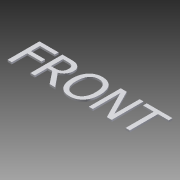
# Autodesk Inventor part: FrontLabel
Saved by Autodesk Inventor 2012 (Build 160160000, 160)
## iProperties
Created: 2014-07-21
Part Number: FrontLabel
Material: Default
Document SubType Name: Modeling
Designer: Anon
Density: 1 g/cm^3
Author: Anon
Autodesk Inventor part; units mm, degrees
ref_plane "YZ Plane" through (0, 0, 0) normal (1, 0, 0) x (0, 1, 0)
ref_plane "XZ Plane" through (0, 0, 0) normal (0, 1, 0) x (-1, 0, 0)
ref_plane "XY Plane" through (0, 0, 0) normal (0, 0, 1) x (1, 0, 0)
sketch "Sketch1" plane through (0, 0, 0) normal (0, 0, 1) x (1, 0, 0)
  line L0 (-12.3971, 6.4501) -> (24.1995, 6.4501) construction
  line L1 (24.1995, 6.4501) -> (24.1995, -12.763) construction
  line L2 (24.1995, -12.763) -> (-12.3971, -12.763) construction
  line L3 (-12.3971, -12.763) -> (-12.3971, 6.4501) construction
  line L4 (-9.9493, 5.9623) -> (-11.5774, 5.9623)
  line L5 (-11.5774, 5.9623) -> (-11.5774, 4.9753)
  line L6 (-11.5774, 4.9753) -> (-10.0174, 4.9753)
  line L7 (-10.0174, 4.9753) -> (-10.0174, 4.5612)
  line L8 (-10.0174, 4.5612) -> (-11.5774, 4.5612)
  line L9 (-11.5774, 4.5612) -> (-11.5774, 2.8764)
  line L10 (-11.5774, 2.8764) -> (-12.0425, 2.8764)
  line L11 (-12.0425, 2.8764) -> (-12.0425, 6.3764)
  line L12 (-12.0425, 6.3764) -> (-9.9493, 6.3764)
  line L13 (-9.9493, 6.3764) -> (-9.9493, 5.9623)
  line L14 (-6.8237, 2.8764) -> (-7.4279, 2.8764)
  line L15 (-7.4279, 2.8764) -> (-8.534, 4.269)
  line L16 (-8.534, 4.269) -> (-9.0673, 4.269)
  line L17 (-9.0673, 4.269) -> (-9.0673, 2.8764)
  line L18 (-9.0673, 2.8764) -> (-9.5324, 2.8764)
  line L19 (-9.5324, 2.8764) -> (-9.5324, 6.3764)
  line L20 (-9.5324, 6.3764) -> (-8.6305, 6.3764)
  spline S0 degree 2 poles (-8.6305, 6.3764) (-8.3298, 6.3764) (-7.9242, 6.3112) (-7.7399, 6.192) knots 0 0 0 1 2 2 2
  spline S1 degree 2 poles (-7.7399, 6.192) (-7.5555, 6.0729) (-7.3428, 5.7014) (-7.3428, 5.4262) knots 0 0 0 1 2 2 2
  spline S2 degree 2 poles (-7.3428, 5.4262) (-7.3428, 5.0433) (-7.7342, 4.5243) (-8.0689, 4.3995) knots 0 0 0 1 2 2 2
  line L21 (-8.0689, 4.3995) -> (-6.8237, 2.8764)
  spline S3 degree 2 poles (-7.8278, 5.3894) (-7.8278, 5.5425) (-7.9356, 5.7779) (-8.049, 5.8545) knots 0 0 0 1 2 2 2
  spline S4 degree 2 poles (-8.049, 5.8545) (-8.1483, 5.9197) (-8.4121, 5.9736) (-8.6049, 5.9736) knots 0 0 0 1 2 2 2
  line L22 (-8.6049, 5.9736) -> (-9.0673, 5.9736)
  line L23 (-9.0673, 5.9736) -> (-9.0673, 4.6576)
  line L24 (-9.0673, 4.6576) -> (-8.6588, 4.6576)
  spline S5 degree 2 poles (-8.6588, 4.6576) (-8.4574, 4.6576) (-8.1369, 4.7285) (-8.0263, 4.8391) knots 0 0 0 1 2 2 2
  spline S6 degree 2 poles (-8.0263, 4.8391) (-7.9242, 4.9356) (-7.8278, 5.2078) (-7.8278, 5.3894) knots 0 0 0 1 2 2 2
  spline S7 degree 2 poles (-4.0697, 5.9765) (-3.8711, 5.7439) (-3.6499, 5.0632) (-3.6499, 4.6264) knots 0 0 0 1 2 2 2
  spline S8 degree 2 poles (-3.6499, 4.6264) (-3.6499, 4.2009) (-3.8655, 3.5117) (-4.0697, 3.2791) knots 0 0 0 1 2 2 2
  spline S9 degree 2 poles (-4.0697, 3.2791) (-4.2852, 3.0352) (-4.8553, 2.8026) (-5.1985, 2.8026) knots 0 0 0 1 2 2 2
  spline S10 degree 2 poles (-5.1985, 2.8026) (-5.5531, 2.8026) (-6.1203, 3.0437) (-6.3274, 3.2791) knots 0 0 0 1 2 2 2
  spline S11 degree 2 poles (-6.3274, 3.2791) (-6.5288, 3.5117) (-6.7443, 4.1953) (-6.7443, 4.6264) knots 0 0 0 1 2 2 2
  spline S12 degree 2 poles (-6.7443, 4.6264) (-6.7443, 5.066) (-6.5259, 5.7354) (-6.3245, 5.9765) knots 0 0 0 1 2 2 2
  spline S13 degree 2 poles (-6.3245, 5.9765) (-6.1203, 6.2091) (-5.5502, 6.4501) (-5.1985, 6.4501) knots 0 0 0 1 2 2 2
  spline S14 degree 2 poles (-5.1985, 6.4501) (-4.8412, 6.4501) (-4.2682, 6.2005) (-4.0697, 5.9765) knots 0 0 0 1 2 2 2
  spline S15 degree 2 poles (-4.1349, 4.6264) (-4.1349, 4.9724) (-4.2852, 5.5085) (-4.4214, 5.6843) knots 0 0 0 1 2 2 2
  spline S16 degree 2 poles (-4.4214, 5.6843) (-4.5604, 5.8659) (-4.9518, 6.0474) (-5.1957, 6.0474) knots 0 0 0 1 2 2 2
  spline S17 degree 2 poles (-5.1957, 6.0474) (-5.4481, 6.0474) (-5.8282, 5.8715) (-5.9728, 5.6843) knots 0 0 0 1 2 2 2
  spline S18 degree 2 poles (-5.9728, 5.6843) (-6.1118, 5.5056) (-6.2593, 4.9667) (-6.2593, 4.6264) knots 0 0 0 1 2 2 2
  spline S19 degree 2 poles (-6.2593, 4.6264) (-6.2593, 3.9372) (-5.6807, 3.2054) (-5.1957, 3.2054) knots 0 0 0 1 2 2 2
  spline S20 degree 2 poles (-5.1957, 3.2054) (-4.7107, 3.2054) (-4.1349, 3.9372) (-4.1349, 4.6264) knots 0 0 0 1 2 2 2
  line L25 (-0.6349, 2.8764) -> (-1.1568, 2.8764)
  line L26 (-1.1568, 2.8764) -> (-2.7054, 5.8942)
  line L27 (-2.7054, 5.8942) -> (-2.7054, 2.8764)
  line L28 (-2.7054, 2.8764) -> (-3.1394, 2.8764)
  line L29 (-3.1394, 2.8764) -> (-3.1394, 6.3764)
  line L30 (-3.1394, 6.3764) -> (-2.4785, 6.3764)
  line L31 (-2.4785, 6.3764) -> (-1.0689, 3.6053)
  line L32 (-1.0689, 3.6053) -> (-1.0689, 6.3764)
  line L33 (-1.0689, 6.3764) -> (-0.6349, 6.3764)
  line L34 (-0.6349, 6.3764) -> (-0.6349, 2.8764)
  line L35 (0.891, 2.8764) -> (0.891, 5.9623)
  line L36 (0.891, 5.9623) -> (-0.2832, 5.9623)
  line L37 (-0.2832, 5.9623) -> (-0.2832, 6.3764)
  line L38 (-0.2832, 6.3764) -> (2.5304, 6.3764)
  line L39 (2.5304, 6.3764) -> (2.5304, 5.9623)
  line L40 (2.5304, 5.9623) -> (1.3562, 5.9623)
  line L41 (1.3562, 5.9623) -> (1.3562, 2.8764)
  line L42 (1.3562, 2.8764) -> (0.891, 2.8764)
  point P0 (0, 0)
  constraints: 2 other
extrude "FrontLabel" add sketch "Sketch1" along normal blind 0.2
body "Solid1"
